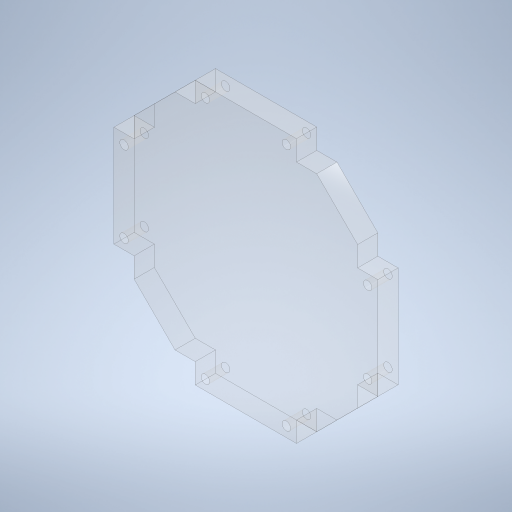
# Autodesk Inventor part: gearbox_top
Saved by Autodesk Inventor 2023 (Build 270158000, 158)
## iProperties
Created: 2023-05-27
Part Number: gearbox_top
Material: PMMA Plastic
Document SubType Name: Modeling
Designer: 310611102
Density: 1.1367 g/cm^3
Appearance: Polycarbonate - Clear
Vendor: 新采硯
Mass: 150.7 g
Surface Area: 323.13 cm^2
Volume: 132.576 cm^3
Author: 310611102
Autodesk Inventor part; units mm, degrees
ref_plane "YZ Plane" through (0, 0, 0) normal (1, 0, 0) x (0, 1, 0)
ref_plane "XZ Plane" through (0, 0, 0) normal (0, 1, 0) x (-1, 0, 0)
ref_plane "XY Plane" through (0, 0, 0) normal (0, 0, 1) x (1, 0, 0)
sketch "Sketch1" plane through (0, 0, 0) normal (0, 0, 1) x (1, 0, 0)
  line L0 (-25, 65.19) -> (25, 65.19)
  line L1 (65.19, 25) -> (65.19, -25)
  line L2 (25, -65.19) -> (-25, -65.19)
  line L3 (-65.19, -25) -> (-65.19, 25)
  line L4 (-50.6308, 50.6308) -> (50.6308, -50.6308) construction
  line L5 (50, 50) -> (-50, -50) construction
  line L6 (-40, 40) -> (-50.6308, 50.6308) construction
  line L7 (-25, 65.19) -> (-25, 55.19)
  line L8 (-25, 55.19) -> (-55.19, 55.19)
  line L9 (-55.19, 55.19) -> (-55.19, 25)
  line L10 (-55.19, 25) -> (-65.19, 25)
  line L11 (-55.19, -25) -> (-55.19, -55.19)
  line L12 (-65.19, -25) -> (-55.19, -25)
  line L13 (-55.19, -55.19) -> (-25, -55.19)
  line L14 (-25, -55.19) -> (-25, -65.19)
  line L15 (-40, -40) -> (-50.6308, -50.6308) construction
  line L16 (25, -55.19) -> (55.19, -55.19)
  line L17 (25, -65.19) -> (25, -55.19)
  line L18 (55.19, -55.19) -> (55.19, -25)
  line L19 (55.19, -25) -> (65.19, -25)
  line L20 (40, -40) -> (50.6308, -50.6308) construction
  line L21 (55.19, 25) -> (55.19, 55.19)
  line L22 (65.19, 25) -> (55.19, 25)
  line L23 (55.19, 55.19) -> (25, 55.19)
  line L24 (25, 55.19) -> (25, 65.19)
  line L25 (40, 40) -> (50.6308, 50.6308) construction
  line L26 (0, 0) -> (0, 26.4544)
  point P0 (-45.3154, 45.3154)
  point P1 (-45.3154, -45.3154)
  point P2 (45.3154, -45.3154)
  point P3 (45.3154, 45.3154)
  dimension "d9" = 130.38
  dimension "d17" = 360
  dimension "d19" = 10
  dimension "d24" = 10
  dimension "d39" = 50
  constraints: 54 end point, 6 coincident, 4 perpendicular, 3 midpoint, 2 parallel, 2 vertical, 1 horizontal, 1 point on line, 54 other
  measures "d9" distance between parallel lines of L2 L0
  measures "d19" distance of L0.start L7.end
  measures "d24" distance of L9.end L3.end
  measures "d39" distance of L0.start L0.end
extrude "Extrusion1" add sketch "Sketch1" along normal blind 10
chamfer "Chamfer1" distance 20.19 angle 45 4 edges at (-55.19, 55.19, 5) (55.19, 55.19, 5) (55.19, -55.19, 5) (-55.19, -55.19, 5)
sketch "Sketch3" plane through (0, 0, 10) normal (0, 0, 1) x (1, 0, 0)
  circle A0 centre (-20, 60.19) radius 2.1
  line L0 (25, 65.19) -> (-25, 65.19) projected
  line L1 (-25, 65.19) -> (-25, 55.19) projected
  line L2 (0, 0) -> (0, 11.031)
  line L3 (0, 0) -> (10.2151, 0)
  circle A1 centre (20, 60.19) radius 2.1
  circle A2 centre (-60.19, -20) radius 2.1
  circle A3 centre (-60.19, 20) radius 2.1
  circle A4 centre (20, -60.19) radius 2.1
  circle A5 centre (-20, -60.19) radius 2.1
  circle A6 centre (60.19, 20) radius 2.1
  circle A7 centre (60.19, -20) radius 2.1
  dimension "d30" = 4.2
  dimension "d31" = 5
  dimension "d32" = 5
  dimension "d35" = 360
  constraints: 8 centre point, 4 end point, 1 horizontal, 1 symmetric about line, 1 vertical, 18 other
  measures "d30" diameter of A0
  measures "d31" distance from line of L0 A0.centre
  measures "d32" distance from line of L1 A0.centre
extrude "Extrusion3" cut sketch "Sketch3" against normal through all
body "Solid1"
